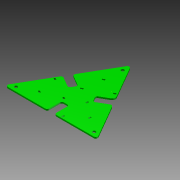
# Autodesk Inventor part: base
Saved by Autodesk Inventor 2012 (Build 160160000, 160)
## iProperties
Created: 2013-10-01
Part Number: base
Material: Default
Document SubType Name: Modeling
Designer: Nick
Density: 1 g/cm^3
Author: Nick
Autodesk Inventor part; units mm, degrees
ref_plane "YZ Plane" through (0, 0, 0) normal (1, 0, 0) x (0, 1, 0)
ref_plane "XZ Plane" through (0, 0, 0) normal (0, 1, 0) x (-1, 0, 0)
ref_plane "XY Plane" through (0, 0, 0) normal (0, 0, 1) x (1, 0, 0)
sketch "Sketch1" plane through (0, 0, 0) normal (0, 0, 1) x (1, 0, 0)
  line L0 (68.7158, -98.8819) -> (-121.2842, -98.8819) construction
  line L1 (-121.2842, -98.8819) -> (-26.2842, 65.663) construction
  line L2 (-26.2842, 65.663) -> (-26.2842, -98.8819) construction
  line L3 (68.7158, -98.8819) -> (-73.7842, -16.6094) construction
  line L4 (-33.7842, -98.8819) -> (-33.7842, -68.8819)
  line L5 (-33.7842, -68.8819) -> (-18.7842, -68.8819)
  line L6 (-18.7842, -68.8819) -> (-18.7842, -98.8819)
  line L7 (-70.0342, -10.1143) -> (-44.0535, -25.1143)
  line L8 (-44.0535, -25.1143) -> (-51.5535, -38.1046)
  line L9 (-51.5535, -38.1046) -> (-77.5342, -23.1046)
  line L10 (-77.5342, -23.1046) -> (-121.2842, -98.8819)
  line L11 (-33.7842, -98.8819) -> (-121.2842, -98.8819)
  line L12 (-18.7842, -98.8819) -> (68.7158, -98.8819)
  line L13 (-26.2842, 65.663) -> (-70.0342, -10.1143)
  line L14 (-121.2842, -98.8819) -> (17.4658, -18.7745) construction
  line L15 (-26.2842, 65.663) -> (68.7158, -98.8819) construction
  line L16 (17.4658, -10.1143) -> (-8.515, -25.1143)
  line L17 (-8.515, -25.1143) -> (-1.015, -38.1046)
  line L18 (-1.015, -38.1046) -> (24.9658, -23.1046)
  line L19 (-26.2842, 65.663) -> (17.4658, -10.1143)
  line L20 (24.9658, -23.1046) -> (68.7158, -98.8819)
  point P0 (-26.2842, -44.0336)
  point P1 (-26.2842, -44.0336)
  dimension "d3" = 190
  dimension "d6" = 7.5
  dimension "d7" = 15
  dimension "d8" = 30
  dimension "d9" = 15
  dimension "d10" = 7.5
  dimension "d16" = 30
  dimension "d18" = 15
  dimension "d19" = 7.5
  dimension "d20" = 30
  constraints: 42 end point, 11 perpendicular, 6 point on line, 3 collinear, 2 midpoint, 2 parallel, 1 coincident, 1 horizontal, 5 other
  measures "d3" distance of L1.end L0.start
  measures "d6" distance between parallel lines of L7 L3
  measures "d7" distance between parallel lines of L7 L9
  measures "d8" distance of L7.start L7.end
  measures "d9" distance of L4.end L5.end
  measures "d10" distance between parallel lines of L4 L2
  measures "d16" distance of L5.end L6.end
  measures "d18" distance of L16.end L17.end
  measures "d19" distance between parallel lines of L16 L14
  measures "d20" distance of L17.end L18.end
extrude "Extrusion2" add sketch "Sketch1" along normal blind 3
fillet "Fillet1" radius 6.75 1 edges at (17.4658, -10.1143, 1.5)
fillet "Fillet2" radius 4 14 edges at (-8.515, -25.1143, 1.5) (24.9658, -23.1046, 1.5) (-1.015, -38.1046, 1.5) (-33.7842, -98.8819, 1.5) (-33.7842, -68.8819, 1.5) (-18.7842, -98.8819, 1.5) (68.7158, -98.8819, 1.5) (-18.7842, -68.8819, 1.5) (-121.2842, -98.8819, 1.5) (-70.0342, -10.1143, 1.5) (-44.0535, -25.1143, 1.5) (-51.5535, -38.1046, 1.5) (-77.5342, -23.1046, 1.5) (-26.2842, 65.663, 1.5)
sketch "Sketch3" plane through (0, 0, 3) normal (0, 0, 1) x (1, 0, 0)
  line L0 (61.7876, -98.8819) -> (-14.7842, -98.8819) projected
  line L1 (-7.2842, -91.8819) -> (-4.2842, -91.8819)
  line L2 (-4.2842, -91.8819) -> (-4.2842, -96.8819)
  line L3 (-4.2842, -96.8819) -> (-7.2842, -96.8819)
  line L4 (-7.2842, -96.8819) -> (-7.2842, -91.8819)
  line L5 (-18.7842, -94.8819) -> (-18.7842, -72.8819) projected
  line L6 (-7.2842, -42.3819) -> (-4.2842, -42.3819)
  line L7 (-4.2842, -42.3819) -> (-4.2842, -47.3819)
  line L8 (-4.2842, -47.3819) -> (-7.2842, -47.3819)
  line L9 (-7.2842, -47.3819) -> (-7.2842, -42.3819)
  line L10 (-74.0701, -25.1046) -> (-55.0176, -36.1046) projected
  line L11 (-117.8201, -92.8819) -> (-79.5342, -26.5687) projected
  line L12 (11.6201, -13.4893) -> (-5.0509, -23.1143) projected
  line L13 (-22.8201, 59.663) -> (14.0908, -4.2686) projected
  line L14 (-34.3845, -23.3069) -> (-32.8845, -25.905)
  line L15 (-32.8845, -25.905) -> (-37.2146, -28.405)
  line L16 (-37.2146, -28.405) -> (-38.7146, -25.8069)
  line L17 (-38.7146, -25.8069) -> (-34.3845, -23.3069)
  line L18 (8.4837, 1.4431) -> (9.9837, -1.155)
  line L19 (9.9837, -1.155) -> (5.6536, -3.655)
  line L20 (5.6536, -3.655) -> (4.1536, -1.0569)
  line L21 (4.1536, -1.0569) -> (8.4837, 1.4431)
  line L22 (-40.1839, -61.412) -> (-38.6839, -58.8139)
  line L23 (-38.6839, -58.8139) -> (-34.3538, -61.3139)
  line L24 (-34.3538, -61.3139) -> (-35.8538, -63.912)
  line L25 (-35.8538, -63.912) -> (-40.1839, -61.412)
  line L26 (-83.0522, -36.662) -> (-81.5522, -34.0639)
  line L27 (-81.5522, -34.0639) -> (-77.222, -36.5639)
  line L28 (-77.222, -36.5639) -> (-78.722, -39.162)
  line L29 (-78.722, -39.162) -> (-83.0522, -36.662)
  line L30 (22.7158, -67.1319) -> (25.7158, -67.1319)
  line L31 (25.7158, -67.1319) -> (25.7158, -72.1319)
  line L32 (25.7158, -72.1319) -> (22.7158, -72.1319)
  line L33 (22.7158, -72.1319) -> (22.7158, -67.1319)
  line L34 (-49.5535, -34.6405) -> (-46.0535, -28.5784) projected
  line L35 (-6.515, -28.5784) -> (-3.015, -34.6405) projected
  line L36 (-30.7805, 9.9508) -> (-32.2805, 12.5489)
  line L37 (-32.2805, 12.5489) -> (-27.9504, 15.0489)
  line L38 (-27.9504, 15.0489) -> (-26.4504, 12.4508)
  line L39 (-26.4504, 12.4508) -> (-30.7805, 9.9508)
  line L40 (-75.118, -72.4197) -> (-76.618, -75.0178)
  line L41 (-76.618, -75.0178) -> (-72.2879, -77.5178)
  line L42 (-72.2879, -77.5178) -> (-70.7879, -74.9197)
  line L43 (-70.7879, -74.9197) -> (-75.118, -72.4197)
  line L44 (-68.0342, -6.6502) -> (-29.7483, 59.663) projected
  line L45 (-47.5176, -23.1143) -> (-66.5701, -12.1143) projected
  line L46 (26.9658, -26.5687) -> (65.2517, -92.8819) projected
  line L47 (-61.1393, 5.2922) -> (-129.5703, -113.2338) construction
  line L48 (-129.5703, -98.8819) -> (82.7932, -98.8819) construction
  line L49 (71.7222, -104.0892) -> (-26.7217, 66.4208) construction
  line L50 (-61.1393, 5.2922) -> (-24.7647, 68.2948) construction
  line L51 (-26.2842, 65.663) -> (-26.2842, -98.8819) construction
  line L52 (68.7158, -98.8819) -> (-73.7842, -16.6094) construction
  line L53 (-121.2842, -98.8819) -> (21.2158, -16.6094) construction
  circle A0 centre (-26.2842, -44.0336) radius 92.5 construction
  circle A1 centre (53.8231, -90.2836) radius 3.175
  circle A2 centre (-106.3916, -90.2836) radius 3.175
  circle A3 centre (-26.2842, 48.4664) radius 3.175
  point P0 (0, 0)
  dimension "d35" = 3
  dimension "d36" = 5
  dimension "d38" = 2
  dimension "d41" = 11.5
  dimension "d42" = 3
  dimension "d43" = 5
  dimension "d44" = 44.5
  dimension "d45" = 3
  dimension "d46" = 5
  dimension "d47" = 3
  dimension "d48" = 5
  dimension "d49" = 44.5
  dimension "d50" = 3
  dimension "d51" = 5
  dimension "d52" = 3
  dimension "d53" = 5
  dimension "d54" = 44.5
  dimension "d55" = 2
  dimension "d56" = 11.5
  dimension "d57" = 11.5
  dimension "d58" = 2
  dimension "d59" = 3
  dimension "d60" = 5
  dimension "d61" = 19.75
  dimension "d62" = 30
  dimension "d63" = 5
  dimension "d64" = 3
  dimension "d65" = 30
  dimension "d66" = 19.75
  dimension "d67" = 3
  dimension "d68" = 5
  dimension "d69" = 19.75
  dimension "d70" = 30
  dimension "d72" = 185
  dimension "d73" = 6.35
  dimension "d74" = 6.35
  dimension "d75" = 6.35
  constraints: 86 end point, 17 parallel, 17 point on line, 12 perpendicular, 4 centre point, 3 horizontal, 3 point on circle, 1 collinear, 1 vertical alignment
  measures "d35" distance of L2.end L3.end
  measures "d36" distance of L1.end L2.end
  measures "d38" distance between parallel lines of L3 L0
  measures "d41" distance between parallel lines of L5 L4
  measures "d42" distance of L7.end L8.end
  measures "d43" distance of L6.end L7.end
  measures "d44" distance between parallel lines of L8 L1
  measures "d45" distance of L15.end L16.end
  measures "d46" distance of L14.end L15.end
  measures "d47" distance of L20.start L20.end
  measures "d48" distance of L18.end L20.start
  measures "d49" distance between parallel lines of L20 L14
  measures "d50" distance of L23.end L24.end
  measures "d51" distance of L22.end L23.end
  measures "d52" distance of L28.start L28.end
  measures "d53" distance of L26.end L28.start
  measures "d54" distance between parallel lines of L28 L22
  measures "d55" distance between parallel lines of L13 L18
  measures "d56" distance between parallel lines of L12 L19
  measures "d57" distance between parallel lines of L10 L27
  measures "d58" distance between parallel lines of L11 L26
  measures "d59" distance of L31.end L32.end
  measures "d60" distance of L30.end L31.end
  measures "d61" distance between parallel lines of L32 L1
  measures "d62" distance between parallel lines of L33 L9
  measures "d63" distance of L36.end L37.end
  measures "d64" distance of L36.start L36.end
  measures "d65" distance between parallel lines of L15 L39
  measures "d66" distance between parallel lines of L36 L14
  measures "d67" distance of L40.start L40.end
  measures "d68" distance of L41.end L40.end
  measures "d69" distance between parallel lines of L40 L28
  measures "d70" distance between parallel lines of L27 L43
  measures "d72" diameter of A0
  measures "d73" diameter of A1
  measures "d74" diameter of A2
  measures "d75" diameter of A3
extrude "Extrusion4" cut sketch "Sketch3" against normal blind 3
equation "\"d6\" = 0.5 * d7"
equation "\"d9\" = d7"
equation "\"d10\" = d6"
equation "\"d16\" = d15"
equation "\"d18\" = d7"
equation "\"d19\" = d6"
equation "\"d20\" = d16"
equation "\"d55\" = d38"
equation "\"d56\" = d41"
equation "\"d57\" = d56"
equation "\"d58\" = d38"
equation "\"d61\" = 0.5 * d44 - 0.5 * d60"
equation "\"d65\" = d62"
equation "\"d66\" = d61"
equation "\"d69\" = d61"
equation "\"d70\" = d62"
equation "\"d15\" = d8"
body "Solid2"
